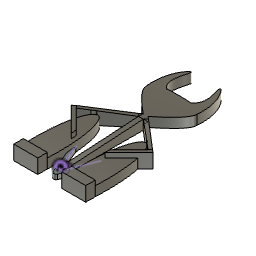
demon (Autodesk Fusion 360 design; units mm, degrees)
Autodesk Fusion 360 part; units mm, degrees
note: some values were not read from the file. Set by a fixed rule: which sketch regions a step uses.
sketch "Sketch1" plane through (0, 0, 0) normal (0, 0, 1) x (1, 0, 0)
  line L0 (-9, 0) -> (-4, 0)
  line L1 (-4, 0) -> (-4, 2)
  line L2 (-4, 2) -> (-9, 2)
  line L3 (-9, 2) -> (-9, 0)
  line L4 (-9, 2) -> (-6.5, 2)
  line L5 (-6.5, 2) -> (-6.5, 15.014)
  spline S0 degree 5 poles (-9, 2) (-9.0171, 2.421) (-9.0441, 3.251) (-9.063, 4.4605) (-9.045, 6.0016) (-8.9496, 7.8046) (-8.7812, 9.475) (-8.5409, 10.9963) (-8.2321, 12.3431) (-7.8609, 13.4798) (-7.4381, 14.3571) (-6.9786, 14.9167) (-6.5, 15.1105) (-6.0214, 14.9167) (-5.5619, 14.3571) (-5.1391, 13.4798) (-4.7679, 12.3431) (-4.4591, 10.9963) (-4.2188, 9.475) (-4.0504, 7.8046) (-3.955, 6.0016) (-3.937, 4.4605) (-3.9559, 3.251) (-3.9829, 2.421) (-4, 2) knots 0 0 0 0 0 0 0.05 0.1 0.15 0.2 0.25 0.3 0.35 0.4 0.45 0.5 0.55 0.6 0.65 0.7 0.75 0.8 0.85 0.9 0.95 1 1 1 1 1 1
  line L6 (-9, 2) -> (-6.5, 2)
  line L7 (-4, 2) -> (-9, 2)
  line L8 (-9, 2) -> (-9, 0)
  spline S1 degree 5 poles (-9, 2) (-9.0171, 2.421) (-9.0441, 3.251) (-9.063, 4.4605) (-9.045, 6.0016) (-8.9496, 7.8046) (-8.7812, 9.475) (-8.5409, 10.9963) (-8.2321, 12.3431) (-7.8609, 13.4798) (-7.4381, 14.3571) (-6.9786, 14.9167) (-6.5, 15.1105) (-6.0214, 14.9167) (-5.5619, 14.3571) (-5.1391, 13.4798) (-4.7679, 12.3431) (-4.4591, 10.9963) (-4.2188, 9.475) (-4.0504, 7.8046) (-3.955, 6.0016) (-3.937, 4.4605) (-3.9559, 3.251) (-3.9829, 2.421) (-4, 2) knots 0 0 0 0 0 0 0.05 0.1 0.15 0.2 0.25 0.3 0.35 0.4 0.45 0.5 0.55 0.6 0.65 0.7 0.75 0.8 0.85 0.9 0.95 1 1 1 1 1 1
  line L9 (-4, 0) -> (-4, 2)
  line L10 (-6.5, 2) -> (-6.5, 15.014)
  line L11 (-9, 0) -> (-4, 0)
  line L12 (3.5, 2) -> (3.5, 15.014)
  line L13 (6, 0) -> (6, 2)
  line L14 (1, 2) -> (3.5, 2)
  line L15 (1, 0) -> (6, 0)
  line L16 (6, 2) -> (1, 2)
  line L17 (3.5, 2) -> (3.5, 15.014)
  line L18 (1, 2) -> (1, 0)
  line L19 (1, 2) -> (1, 0)
  line L20 (6, 2) -> (1, 2)
  line L21 (1, 2) -> (3.5, 2)
  spline S2 degree 5 poles (1, 2) (0.9829, 2.421) (0.9559, 3.251) (0.937, 4.4605) (0.955, 6.0016) (1.0504, 7.8046) (1.2188, 9.475) (1.4591, 10.9963) (1.7679, 12.3431) (2.1391, 13.4798) (2.5619, 14.3571) (3.0214, 14.9167) (3.5, 15.1105) (3.9786, 14.9167) (4.4381, 14.3571) (4.8609, 13.4798) (5.2321, 12.3431) (5.5409, 10.9963) (5.7812, 9.475) (5.9496, 7.8046) (6.045, 6.0016) (6.063, 4.4605) (6.0441, 3.251) (6.0171, 2.421) (6, 2) knots 0 0 0 0 0 0 0.05 0.1 0.15 0.2 0.25 0.3 0.35 0.4 0.45 0.5 0.55 0.6 0.65 0.7 0.75 0.8 0.85 0.9 0.95 1 1 1 1 1 1
  spline S3 degree 5 poles (1, 2) (0.9829, 2.421) (0.9559, 3.251) (0.937, 4.4605) (0.955, 6.0016) (1.0504, 7.8046) (1.2188, 9.475) (1.4591, 10.9963) (1.7679, 12.3431) (2.1391, 13.4798) (2.5619, 14.3571) (3.0214, 14.9167) (3.5, 15.1105) (3.9786, 14.9167) (4.4381, 14.3571) (4.8609, 13.4798) (5.2321, 12.3431) (5.5409, 10.9963) (5.7812, 9.475) (5.9496, 7.8046) (6.045, 6.0016) (6.063, 4.4605) (6.0441, 3.251) (6.0171, 2.421) (6, 2) knots 0 0 0 0 0 0 0.05 0.1 0.15 0.2 0.25 0.3 0.35 0.4 0.45 0.5 0.55 0.6 0.65 0.7 0.75 0.8 0.85 0.9 0.95 1 1 1 1 1 1
  line L22 (6, 0) -> (6, 2)
  line L23 (1, 0) -> (6, 0)
  line L24 (-1.4961, 0) -> (-1.4961, 1.0146)
  line L25 (-2, 1.5) -> (-2, 20)
  line L26 (-2, 20) -> (-1, 20)
  line L27 (-1, 20) -> (-1, 1.6145)
  spline S4 degree 5 poles (-1, 20) (-0.5781, 20.3374) (0.2186, 20.9908) (1.2723, 21.9063) (2.3934, 22.9976) (3.3182, 24.1444) (3.7672, 25.0744) (3.752, 25.7935) (3.3004, 26.3149) (2.4649, 26.6641) (1.3224, 26.8757) (-0.034, 26.9841) (-1.5, 27.0163) (-2.966, 26.9841) (-4.3224, 26.8757) (-5.4649, 26.6641) (-6.3004, 26.3149) (-6.752, 25.7935) (-6.7672, 25.0744) (-6.3182, 24.1444) (-5.3934, 22.9976) (-4.2723, 21.9063) (-3.2186, 20.9908) (-2.4219, 20.3374) (-2, 20) knots 0 0 0 0 0 0 0.05 0.1 0.15 0.2 0.25 0.3 0.35 0.4 0.45 0.5 0.55 0.6 0.65 0.7 0.75 0.8 0.85 0.9 0.95 1 1 1 1 1 1
  spline S5 degree 5 poles (-6.6986, 25.498) (-6.7188, 25.7145) (-6.7501, 26.1428) (-6.7702, 26.7715) (-6.7426, 27.5821) (-6.6181, 28.5468) (-6.4072, 29.4568) (-6.1189, 30.3009) (-5.7703, 31.0608) (-5.3885, 31.7102) (-5.0149, 32.2118) (-4.7033, 32.5197) (-4.5022, 32.5952) (-4.4417, 32.4187) (-4.5135, 32.0077) (-4.6759, 31.4125) (-4.8699, 30.6991) (-5.0311, 29.9377) (-5.1043, 29.1885) (-5.0553, 28.4898) (-4.8654, 27.8635) (-4.5946, 27.4284) (-4.3239, 27.1404) (-4.1136, 26.9653) (-4.0009, 26.882) knots 0 0 0 0 0 0 0.05 0.1 0.15 0.2 0.25 0.3 0.35 0.4 0.45 0.5 0.55 0.6 0.65 0.7 0.75 0.8 0.85 0.9 0.95 1 1 1 1 1 1
  spline S6 degree 5 poles (3.6986, 25.4978) (3.7188, 25.7127) (3.7502, 26.1383) (3.77, 26.7637) (3.7421, 27.5717) (3.6167, 28.5361) (3.4047, 29.4488) (3.115, 30.2981) (2.7649, 31.0653) (2.3817, 31.7232) (2.007, 32.2334) (1.695, 32.5483) (1.494, 32.628) (1.4341, 32.4521) (1.5071, 32.0381) (1.671, 31.4369) (1.8667, 30.7159) (2.0297, 29.9467) (2.1044, 29.1908) (2.0565, 28.4873) (1.867, 27.8589) (1.5959, 27.4242) (1.3247, 27.1378) (1.1139, 26.9644) (1.0009, 26.882) knots 0 0 0 0 0 0 0.05 0.1 0.15 0.2 0.25 0.3 0.35 0.4 0.45 0.5 0.55 0.6 0.65 0.7 0.75 0.8 0.85 0.9 0.95 1 1 1 1 1 1
  line L28 (-1.4961, 0) -> (-3.9769, 6.0828)
  line L29 (-1.4961, 0) -> (0.9762, 6.0622)
  line L30 (-2, 19) -> (-9, 13)
  line L31 (-9, 13) -> (-5, 9)
  line L32 (-5, 9) -> (-5, 8)
  line L33 (-5, 8) -> (-10, 13)
  line L34 (-10, 13) -> (-2, 20)
  line L35 (-1, 19) -> (6, 13)
  line L36 (6, 13) -> (2, 9)
  line L37 (2, 9) -> (2, 8)
  line L38 (2, 8) -> (7, 13)
  line L39 (7, 13) -> (-1, 20)
  line L40 (-1.4961, 1.0146) -> (-1.4961, 1.5)
  line L41 (-1.4961, 1.5) -> (-4.0879, 8.0143)
  line L42 (-1.4961, 1.5) -> (1.0879, 8.0143)
  point P0 (-8, 13)
  point P1 (-5, 13)
  point P2 (-8, 13)
  point P3 (-5, 13)
  point P4 (5, 13)
  point P5 (2, 13)
  point P6 (2, 13)
  point P7 (5, 13)
  point P8 (3.5, 26)
  point P9 (-1.5, 27)
  point P10 (-6.5, 26)
  point P11 (-5.5, 31.5)
  point P12 (-4.5, 32.5)
  point P13 (-5, 30)
  point P14 (2.5, 31.5)
  point P15 (1.492, 32.5325)
  point P16 (2, 30)
  constraint horizontal L0
  constraint perpendicular L0 L1
  constraint perpendicular L1 L2
  constraint perpendicular L0 L3
  constraint horizontal L4
  constraint vertical L5
  constraint horizontal L11
  constraint perpendicular L9 L11
  constraint perpendicular L7 L9
  constraint perpendicular L8 L11
  constraint horizontal L6
  constraint vertical L10
  constraint horizontal L23
  constraint perpendicular L22 L23
  constraint perpendicular L20 L22
  constraint perpendicular L18 L23
  constraint horizontal L14
  constraint vertical L12
  constraint horizontal L15
  constraint perpendicular L13 L15
  constraint perpendicular L13 L16
  constraint perpendicular L15 L19
  constraint horizontal L21
  constraint vertical L17
  constraint vertical L25
  constraint perpendicular L25 L26
  constraint perpendicular L26 L27
  constraint coincident S4 S5.start
  constraint coincident S4 S5.end
  constraint coincident S4 S6.start
  constraint coincident S4 S6.end
  constraint coincident S1 L28.end
  constraint coincident S2 L29.end
  constraint coincident L25 L30.start
  constraint parallel L10 L32
  constraint parallel L31 L33
  constraint coincident L27 L35.start
  constraint parallel L12 L37
  constraint parallel L36 L38
  constraint parallel L24 L40
  constraint coincident S1 L41.end
  constraint coincident S3 L42.end
extrude "Extrude2" add sketch "Sketch1" along normal blind 3 contours L0 L1 L2 L3 L4 L6 L7 L8 L9 L11 | L13 L14 L15 L16 L18 L19 L20 L21 L22 L23 makes body 1 at (-5.6667, 2, 1) makes body 2 at (2.6667, 2, 1)
extrude "Extrude3" add sketch "Sketch1" along normal blind 2 contours L2 L4 L5 S0 L6 L7 S1 L10 L33 | L2 L5 S0 L7 S1 L10 L31 L32 L33 | L5 S0 S1 L10 L30 L31 | L25 L26 L27 L41 L42 | L12 L14 L16 L17 L20 L21 S2 S3 L36 L37 L38 | L12 L16 L17 L20 S2 S3 L38 | L12 L17 S2 S3 L35 L36 bodies 1 2 makes body 3
extrude "Extrude4" add sketch "Sketch1" along normal blind 1 contours S0 S1 L24 L28 L40 L41 | S2 S3 L24 L29 L40 L42 bodies 1 2 3
extrude "Extrude5" add sketch "Sketch1" along normal blind 3 separate body contours S0 S1 L25 L30 L31 L33 L34 | L5 S0 S1 L10 L31 L33 | L5 L10 L31 L32 L33 | S2 S3 L27 L35 L36 L38 L39 | L12 L17 S2 S3 L36 L38 | L12 L17 L36 L37 L38 makes body 4 at (-7.3333, 15.3333, 1) makes body 5 at (4.3333, 15.3333, 1)
extrude "Extrude6" add sketch "Sketch1" along normal blind 2 contours L26 S4 | S4 S5 | S4 S6 bodies 1 4 5
sketch "Sketch3" plane through (-10.2353, 11.9412, 0) normal (0.650791, -0.759257, 0) x (0.759257, 0.650791, 0)
  line L0 (4.6785, 0) -> (10.8465, 0)
  line L1 (10.8465, 0) -> (10.8465, 2)
  line L2 (10.8465, 2) -> (10.8465, 3)
  line L3 (10.8465, 3) -> (4.6785, 3)
  line L4 (4.6785, 3) -> (4.6785, 2)
  line L5 (4.6785, 2) -> (4.6785, 0)
  line L6 (11.5, 2) -> (11.5, 3.1347)
  line L7 (11.5, 3.1347) -> (1.645, 3)
  line L8 (1.645, 3) -> (10.8465, 2)
  line L9 (11.5, 2) -> (10.8465, 2)
  constraint perpendicular L3 L6
  constraint coincident L1.end L2.start
extrude "Extrude7" cut sketch "Sketch3" against normal blind 10 contours L2 L3 L4 L8 | L2 L3 L4 L6 L7 L8 L9 bodies 1
sketch "Sketch4" plane through (8.9647, 10.4588, 0) normal (-0.650791, -0.759257, 0) x (0.759257, -0.650791, 0)
  line L0 (-13.1243, 0) -> (-6.9563, 0)
  line L1 (-6.9563, 0) -> (-6.9563, 2)
  line L2 (-6.9563, 2) -> (-6.9563, 3)
  line L3 (-6.9563, 3) -> (-13.1243, 3)
  line L4 (-13.1243, 3) -> (-13.1243, 2)
  line L5 (-13.1243, 2) -> (-13.1243, 0)
  line L6 (-3.9078, 3.0037) -> (-13.1243, 2)
  line L7 (-13.8877, 2) -> (-13.8877, 3.2682)
  line L8 (-13.8877, 2) -> (-13.1243, 2)
  line L9 (-13.8877, 3.2682) -> (-3.9078, 3.0037)
  constraint coincident L4.end L5.start
  constraint parallel L4 L7
  constraint perpendicular L4 L8
extrude "Extrude8" cut sketch "Sketch4" against normal blind 10 contours L2 L3 L4 L6 L7 L8 L9 | L2 L3 L4 L6 bodies 1
sketch "Sketch5" plane through (-2, 0, 0) normal (-1, 0, 0) x (0, -1, 0)
  line L0 (-19, 2) -> (-19, 0)
  line L1 (-19, 0) -> (-2.7664, 0)
  line L2 (-2.7664, 2) -> (-19, 2)
  line L3 (-19, 2) -> (-2.226, 1)
  line L4 (-2.7664, 2) -> (-19, 2)
  line L5 (-2.226, 1) -> (-1, 1)
  line L6 (-1, 1) -> (-1, 2.2977)
  line L7 (-1, 2.2977) -> (-2.7664, 2)
  line L8 (-2.7664, 0) -> (-2.7664, 1)
  line L9 (-2.7664, 1) -> (-2.7664, 2)
  constraint coincident L0.start L2.end
  constraint coincident L2.start L4.start
  constraint perpendicular L5 L6
extrude "Extrude9" cut sketch "Sketch5" against normal blind 2 contours L2 L3 L4 L9 | L3 L5 L6 L7 L9 bodies 1
sketch "Sketch6" plane through (0, 0, 1) normal (0, 0, 1) x (-1, 0, 0)
  line L0 (1.4961, 0) -> (-0.9762, -6.0622)
  spline S0 degree 3 poles (-1.0879, -8.0143) (-1.0347, -7.3711) (-0.9983, -6.7182) (-0.9762, -6.0622) knots -0.592258 -0.592258 -0.592258 -0.592258 -0.399427 -0.399427 -0.399427 -0.399427
  line L1 (1.2082, -2.226) -> (1.785, -2.226)
  spline S1 degree 3 poles (3.9769, -6.0828) (3.9991, -6.7319) (4.0353, -7.3778) (4.0879, -8.0143) knots -0.240254 -0.240254 -0.240254 -0.240254 -0.050019 -0.050019 -0.050019 -0.050019
  line L2 (3.9769, -6.0828) -> (1.4961, 0)
  line L3 (-1.0879, -8.0143) -> (1, -2.7507)
  line L4 (1, -2.7507) -> (1.2082, -2.226)
  line L5 (1.785, -2.226) -> (2, -2.7664)
  line L6 (2, -2.7664) -> (4.0879, -8.0143)
fillet "Fillet1" radius 0.5 1 edges at (-1.4961, 0, 0.5) on bodies 1
